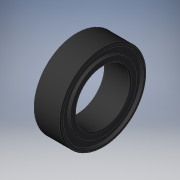
# Autodesk Inventor part: bearing_675
Saved by Autodesk Inventor 2019 (Build 230136000, 136)
## iProperties
Created: 2023-11-09
Part Number: bearing_675
Material: Generic
Catalog Web Link: www.cadenas.de
Description: 600_bearing-Small Ball Bearings
Vendor: MISUMI
Document SubType Name: Modeling
Designer: psAdmin
Manufacturer: MISUMI
Mass: 0.0696167 g
Surface Area: 1.81567 cm^2
Volume: 0.0696167 cm^3
Density: 1 g/cm^3
Appearance: PSOLRGB-175-175-175
Category: PARTsolutions
Company: MISUMI
Title: bearing_675
Author: Cadenas PARTsolutions
Comments: Small Ball Bearings
PSOL_IDENT_0: {$CADENAS_DATA/23d-libs/misumi/metric/accessories/bearing_600.prj},167 {VTYP=3D},{NB=bearing_675},{L
PSOL_IDENT_1: INA=bearing_675},{NN=600_bearing},{DATE=08.06.2021 06:39:28},{GEOMDATE=24.10.2013 00:00:00},{VERSION=
PSOL_IDENT_2: },{LINEID=70},{WBVAR=},{WBNUMERIC=}  {NB=bearing_675},{LINA=bearing_675},{KT=DUMMY},{PN=bearing_675}
PSOL_IDENT_3: ,{BN=675},{DD=5.0},{D=8},{B=2.5},{RR=0.10},{DS=5.80},{DDHH=7.40},{R=0.10},{MASS=0.34},{A=1.9900},{C=
PSOL_IDENT_4: 0.575},{BB=0.300}
NB: bearing_675
NN: 600_bearing
NT: Small Ball Bearings
NBSYN: $PN.
LINA: bearing_675
CATALOG: Misumi
PN: bearing_675
BN: 675
DD: 5
D: 8
B: 2.5
RR: 0.1
DS: 5.8
DDHH: 7.4
R: 0.1
MASS: 0.34
SUPPLIER: MISUMI
ARTICLENO: bearing_675
BOMINFO: bearing_675
CREATOR: CADENAS GmbH
Autodesk Inventor part; units mm, degrees
sketch "Sketch_1" plane through (0, 0, 0) normal (0, 0, 1) x (1, 0, 0)
  line L0 (2.4, 0) -> (0.1, 0)
  arc A0 (0, 2.6) -> (0.1, 2.5) centre (0.1, 2.6) ccw
  line L1 (0.1, 2.5) -> (2.4, 2.5)
  arc A1 (2.4, 2.5) -> (2.5, 2.6) centre (2.4, 2.6) ccw
  line L2 (2.5, 2.6) -> (2.5, 3.075)
  line L3 (2.5, 3.075) -> (2.245, 3.075)
  line L4 (2.245, 3.075) -> (2.245, 3.7)
  line L5 (2.245, 3.7) -> (2.5, 3.7)
  line L6 (2.5, 3.7) -> (2.5, 3.9)
  arc A2 (2.5, 3.9) -> (2.4, 4) centre (2.4, 3.9) ccw
  line L7 (2.4, 4) -> (0.1, 4)
  arc A3 (0.1, 4) -> (0, 3.9) centre (0.1, 3.9) ccw
  line L8 (0, 3.9) -> (0, 3.7)
  line L9 (0, 3.7) -> (0.255, 3.7)
  line L10 (0.255, 3.7) -> (0.255, 3.075)
  line L11 (0.255, 3.075) -> (0, 3.075)
  line L12 (0, 3.075) -> (0, 2.6)
  constraints: 26 end point, 8 point on circle, 4 centre point
revolve "Revolution1" add sketch "Sketch_1" angle 360 about axis through (2.4, 0, 0) along (1, 0, 0)
ref_plane "to_housing_XY" through (0, 0, 0) normal (1, 0, 0) x (0, 0, -1)
ref_plane "to_housing_YZ" through (0, 0, 0) normal (0, 0, -1) x (0, 1, 0)
ref_plane "to_housing_ZX" through (0, 0, 0) normal (0, 1, 0) x (1, 0, 0)
ref_plane "to_housing_center_XY" through (1.25, 0, 0) normal (1, 0, 0) x (0, 0, -1)
ref_plane "to_housing_center_YZ" through (1.25, 0, 0) normal (0, 0, -1) x (0, 1, 0)
ref_plane "to_housing_center_ZX" through (1.25, 0, 0) normal (0, 1, 0) x (1, 0, 0)
body "Solid1"
